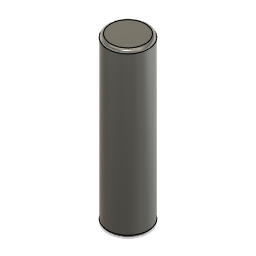
Finger v50 (Autodesk Fusion 360 archive; units mm, degrees)
design "Finger Pin"
Autodesk Fusion 360 part; units mm, degrees
sketch "Sketch1" plane through (0, 0, 0) normal (0, 1, 0) x (1, 0, 0)
  circle A0 centre (0, 0) radius 2
  dimension "d1" = 4
  constraint coincident A0.centre origin
  measures "d1" diameter of A0
extrude "Extrude1" add sketch "Sketch1" along normal blind 16
fillet "Fillet1" radius 0.3 2 edges at (-1.8647, 16, 0.7232) (-1.8647, 0, 0.7232)
